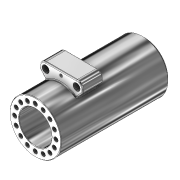
# Autodesk Inventor part: Piston_Housing
Saved by Autodesk Inventor 2020.1 (Build 241239000, 239)
## iProperties
Part Number: Piston_Housing
Document SubType Name: Modeling
Created: 2003-05-03
Designer: Stephen Hooper
Manufacturer: Standard
Standards Organization: Custom
Material: Generic
Density: 1 g/cm^3
Appearance: Black Chrome
Control State: 0
Master: False
Checked Out: False
Shininess: 64.0
Length Units: 11269
Angle Units: 11279
Time Units: 11290
Mass Units: 11283
Length Display Precision: 3
Angle Display Precision: 2
Compacted: True
Density: 0.0
Volumn: 0.0
Area: 0.0
PropertySet Name: Model Information
Author: Stephen Hooper
Autodesk Inventor part; units mm, degrees
ref_plane "YZ Plane" through (0, 0, 0) normal (1, 0, 0) x (0, 1, 0)
ref_plane "XZ Plane" through (0, 0, 0) normal (0, 1, 0) x (-1, 0, 0)
sketch "Sketch1" plane through (0, 0, 0) normal (0, 0, 1) x (1, 0, 0)
  line L0 (0, -50) -> (212, -50)
  line L1 (212, -50) -> (212, 0)
  line L2 (212, 0) -> (197, 0)
  line L3 (197, 0) -> (197, -31.5)
  line L4 (197, -31.5) -> (0, -31.5)
  line L5 (0, -31.5) -> (0, -50)
  point P0 (0, 0)
  dimension "d0" = 50
  dimension "d1" = 212
  dimension "d2" = 15
  dimension "d44" = 31.5
  constraints: 12 end point, 3 parallel, 2 perpendicular, 2 point on line, 1 horizontal
  measures "d0" distance between parallel lines of L2 L0
  measures "d1" distance of L0.start L0.end
  measures "d2" distance of L1.end L2.end
  measures "d44" distance between parallel lines of L2 L4
revolve "Revolution1" add sketch "Sketch1" angle 360 about axis through (212, 0, 0) along (-1, 0, 0)
sketch "Sketch2" plane through (0, 0, 0) normal (-1, 0, 0) x (0, 0, 1)
  circle A0 centre (0, 0) radius 31.5 projected
  point P0 (40, 0)
  dimension "d5" = 40
  constraints: 1 horizontal alignment
  measures "d5" distance of point (40, 0) A0.centre
hole "Hole1" at (0, 0, 40) direction (1, 0, 0) diameter 8.376 depth 30 tip angle 118 thread size "M10x1.5" class "6H" standard "ISO Metric profile"
pattern_circular "Circular Pattern1" count 16 over 360 about axis through (98.5, 0, 0) along (-1, 0, 0) of "Hole1"
chamfer "Chamfer1" distance 1 angle 45 2 edges at (0, 50, 0) (0, 31.5, 0)
chamfer "Chamfer2" distance 5 angle 45 1 edges at (212, 50, 0)
ref_plane "Work Plane1" through (50, 0, 0) normal (-1, 0, 0) x (0, 0, 1)
sketch "Sketch3" plane through (50, 0, 0) normal (-1, 0, 0) x (0, 0, 1)
  circle A0 centre (0, 0) radius 50 projected
  line L0 (0, 0) -> (50, 0) construction
  line L1 (40, 30) -> (40, -30) construction
  line L2 (40, 30) -> (50, 38.9443)
  arc A1 (70, 30) -> (50, 38.9443) centre (58, 30) ccw
  line L3 (70, 30) -> (70, -30)
  arc A2 (50, -38.9443) -> (70, -30) centre (58, -30) ccw
  line L4 (50, -38.9443) -> (40, -30)
  dimension "d21" = 60
  dimension "d22" = 12
  dimension "d23" = 30
  constraints: 10 end point, 7 point on circle, 4 tangent, 2 centre point, 2 horizontal alignment, 1 equal length, 1 equal radius, 1 horizontal, 1 parallel, 1 perpendicular
  measures "d21" distance of L1.start L1.end
  measures "d22" radius of A1
  measures "d23" distance between parallel lines of L1 L3
extrude "Extrusion1" add sketch "Sketch3" against normal blind 40 contours A0 L2 A1 L3 A2 L4
sketch "Sketch4" plane through (50, 0, 0) normal (-1, 0, 0) x (0, 0, 1)
  arc A0 (50, -38.9443) -> (70, -30) centre (58, -30) ccw projected
  arc A1 (70, 30) -> (50, 38.9443) centre (58, 30) ccw projected
  constraints: 2 coincident
hole "Hole2" at (50, -30, 58) at (50, 30, 58) direction (1, 0, 0) diameter 13.835 depth 35 tip angle 118 thread size "M16x2" class "6H" standard "ISO Metric profile"
sketch "Sketch5" plane through (50, 0, 0) normal (-1, 0, 0) x (0, 0, 1)
  line L0 (70, -30) -> (70, 30) projected
  circle A0 centre (58, -30) radius 6.9175 projected
  point P0 (62, 0)
  point P1 (70, 0)
  dimension "d46" = 4
  constraints: 1 horizontal alignment, 1 midpoint
  measures "d46" horizontal distance of point (62, 0) A0.centre
hole "Hole3" at (50, 0, 62) direction (1, 0, 0) diameter 6 depth 35 tip angle 118
fillet "Fillet1" radius 2 10 edges at (50, 0, 70) (50, 40.9545, 62.899) (50, 34.4721, 45) (50, -40.9545, 62.899) (50, -34.4721, 45) (90, -40.9545, 62.899) (90, 0, 70) (90, 40.9545, 62.899) (90, 34.4721, 45) (90, -34.4721, 45)
fillet "Fillet2" radius 2 8 edges at (50, 0, 50) (50.6885, 29.6049, 40.2933) (70, 30, 40) (89.3115, 29.6049, 40.2933) (90, 0, 50) (89.3115, -29.6049, 40.2933) (70, -30, 40) (50.6885, -29.6049, 40.2933)
fillet "Fillet3" radius 1 1 edges at (197, 31.5, 0)
equation "\"d5\" = d0 - 0.5 * d3"
equation "\"d3\" = 20"
body "Solid1"
